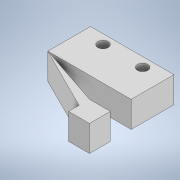
# Autodesk Inventor part: limit_switch
Saved by Autodesk Inventor 2022 (Build 260153000, 153)
## iProperties
Created: 2022-02-08
Part Number: limit_switch
Material: Generic
Document SubType Name: Modeling
Designer: kylem
Density: 1 g/cm^3
Appearance: Default
Author: kylem
Autodesk Inventor part; units mm, degrees
ref_plane "YZ Plane" through (0, 0, 0) normal (1, 0, 0) x (0, 1, 0)
ref_plane "XZ Plane" through (0, 0, 0) normal (0, 1, 0) x (-1, 0, 0)
ref_plane "XY Plane" through (0, 0, 0) normal (0, 0, 1) x (1, 0, 0)
sketch "Sketch1" plane through (0, 0, 0) normal (0, 1, 0) x (-1, 0, 0)
  line L0 (0, 0) -> (20, 0)
  line L1 (20, 0) -> (20, -10.25)
  line L2 (20, -10.25) -> (0, -10.25)
  line L3 (0, -10.25) -> (0, 0)
  dimension "d0" = 20
  dimension "d1" = 10.25
  constraints: 8 end point, 2 parallel, 1 horizontal, 1 perpendicular
  measures "d0" distance of L1.end L2.end
  measures "d1" distance of L0.end L1.end
extrude "Extrusion1" add sketch "Sketch1" along normal blind 6.25
sketch "Sketch2" plane through (0, 0, 0) normal (0, -1, 0) x (1, 0, 0)
  line L0 (-20, 0) -> (0, 0) projected
  line L1 (0, 0) -> (0, 5)
  line L2 (0, 5) -> (-5, 5)
  line L3 (-5, 5) -> (-5, 10)
  line L4 (-5, 10) -> (0, 10)
  line L5 (0, 10) -> (0, 5)
  line L6 (-20, -10.25) -> (-20, 0) projected
  line L7 (-5, 5) -> (-20, 0)
  line L8 (-20, 0) -> (-5, 7.5)
  dimension "d4" = 5
  dimension "d5" = 5
  dimension "d6" = 5
  constraints: 14 end point, 2 parallel, 1 horizontal, 1 midpoint, 1 perpendicular, 1 vertical
  measures "d4" distance of L0.end L1.end
  measures "d5" distance of L3.end L4.end
  measures "d6" distance of L2.end L3.end
extrude "Extrusion2" add sketch "Sketch2" against normal blind 6.25 contours L8 L3 L7 | L3 L4 L5 L2
sketch "Sketch3" plane through (0, 0, 0) normal (0, -1, 0) x (1, 0, 0)
  line L0 (0, -10.25) -> (-20, -10.25) projected
  line L1 (0, -10.25) -> (-5.25, -10.25)
  line L2 (-5.25, -10.25) -> (-5.25, -8)
  line L3 (-5.25, -8) -> (0, -8)
  line L4 (0, -8) -> (0, -10.25)
  line L5 (-20, -10.25) -> (-14.75, -10.25)
  line L6 (-14.75, -10.25) -> (-14.75, -8)
  line L7 (-14.75, -8) -> (-20, -8)
  line L8 (-20, -8) -> (-20, -10.25)
  circle A0 centre (-14.75, -8) radius 1.25
  circle A1 centre (-5.25, -8) radius 1.25
  point P0 (0, 0)
  dimension "d9" = 5.25
  dimension "d10" = 2.25
  dimension "d11" = 5.25
  dimension "d12" = 2.25
  dimension "d13" = 2.5
  dimension "d14" = 2.5
  constraints: 16 end point, 4 parallel, 2 centre point, 2 coincident, 2 horizontal, 2 perpendicular
  measures "d9" distance of L2.end L3.end
  measures "d10" distance of L1.end L2.end
  measures "d11" distance of L7.end L6.end
  measures "d12" distance of L6.end L5.end
  measures "d13" diameter of A0
  measures "d14" diameter of A1
extrude "Extrusion3" cut sketch "Sketch3" against normal blind 6.25 contours A1 L3 L2 | L2 L3 A1 | A0 L7 L6 | L6 L7 A0
body "Solid1"
